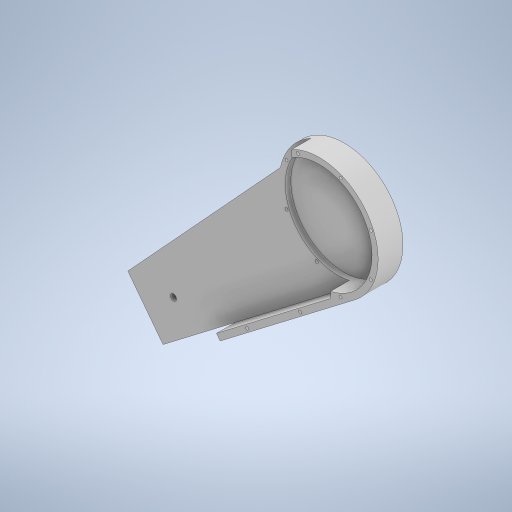
# Autodesk Inventor part: legparts_05
Saved by Autodesk Inventor 2024.3 (Build 283343000, 343)
## iProperties
Created: 2024-10-20
Part Number: legparts_05
Material: 一般
Document SubType Name: Modeling
Designer: 佐藤智貴
Density: 1 g/cm^3
Appearance: 既定
Author: 佐藤智貴
Autodesk Inventor part; units mm, degrees
ref_plane "YZ Plane" through (0, 0, 0) normal (1, 0, 0) x (0, 1, 0)
ref_plane "XZ Plane" through (0, 0, 0) normal (0, 1, 0) x (-1, 0, 0)
ref_plane "XY Plane" through (0, 0, 0) normal (0, 0, 1) x (1, 0, 0)
sketch "スケッチ1" plane through (0, 0, 0) normal (0, 0, 1) x (1, 0, 0)
  circle A0 centre (0, 0) radius 48.5
  circle A1 centre (0, 0) radius 46
  dimension "d0" = 97
  dimension "d1" = 92
  constraints: 2 centre point, 1 coincident
  measures "d0" diameter of A0
  measures "d1" diameter of A1
extrude "押し出し1" add sketch "スケッチ1" along normal blind 20.5 contours A0 | A1
sketch "スケッチ2" plane through (0, 0, 20.5) normal (0, 0, 1) x (1, 0, 0)
  circle A0 centre (0, 0) radius 46
  line L0 (0, 0) -> (0, 59.211017)
  line L1 (0, 0) -> (-21.860946, 52.776992)
  line L2 (0, 0) -> (27.822621, 47.858094)
  point P0 (-17.603438, 42.498458)
  point P1 (-42.498458, 17.603438)
  point P2 (-42.498458, -17.603438)
  point P3 (-17.603438, -42.498458)
  point P4 (17.603438, -42.498458)
  point P5 (42.498458, -17.603438)
  point P6 (42.498458, 17.603438)
  point P7 (17.603438, 42.498458)
  dimension "d4" = 92
  dimension "d5" = 22.5
  dimension "d8" = 360
  constraints: 6 end point, 1 coincident, 1 point on line, 1 vertical, 12 other
  measures "d5" angle of L1 L0
hole "穴1" at (-17.603438, 42.498458, 20.5) at (-42.498458, 17.603438, 20.5) at (-42.498458, -17.603438, 20.5) at (-17.603438, -42.498458, 20.5) at (17.603438, -42.498458, 20.5) at (42.498458, -17.603438, 20.5) at (42.498458, 17.603438, 20.5) at (17.603438, 42.498458, 20.5) direction (0, 0, -1) diameter 2.459 end through all
sketch "スケッチ3" plane through (0, 0, 20.5) normal (0, 0, 1) x (1, 0, 0)
  circle A0 centre (0, 0) radius 43.5
  dimension "d17" = 87
  constraints: 1 centre point, 1 coincident
  measures "d17" diameter of A0
extrude "押し出し2" cut sketch "スケッチ3" against normal blind 20
sketch "スケッチ4" plane through (0, 0, 0) normal (0, 0, -1) x (-1, 0, 0)
  line L0 (0, 0) -> (0, -80.557014)
  circle A0 centre (0, 0) radius 48.5
  line L1 (-29.457728, -38.529109) -> (145.313488, -172.151794)
  line L2 (29.457728, 38.529109) -> (204.228945, -95.093576)
  line L3 (145.313488, -172.151794) -> (204.228945, -95.093576)
  point P0 (29.457728, 38.529109)
  dimension "d21" = 48.5
  dimension "d23" = 97
  dimension "d24" = 220
  dimension "d25" = 220
  dimension "d56" = 52.6
  constraints: 8 end point, 1 perpendicular, 1 vertical, 2 other
  measures "d21" distance from line of L1 L0.start
  measures "d23" distance between parallel lines of L2 L1
  measures "d24" distance of L2.start L2.end
  measures "d25" distance of L1.start L1.end
  measures "d56" angle of L2 L0
extrude "押し出し3" add sketch "スケッチ4" against normal blind 5 contours A0 L2 L3 L1 L0 | L0 L1 A0
sketch "スケッチ5" plane through (0, 0, 5) normal (0, 0, 1) x (1, 0, 0)
  line L0 (-29.457728, 38.529109) -> (29.457728, -38.529109)
  line L1 (-204.228945, -95.093576) -> (-145.313488, -172.151794)
  line L2 (29.457728, -38.529109) -> (-145.313488, -172.151794)
  line L3 (-145.313488, -172.151794) -> (-204.228945, -95.093576)
  line L4 (-204.228945, -95.093576) -> (-29.457728, 38.529109)
  line L5 (-26.420849, 34.557036) -> (-201.192066, -99.065649)
  line L6 (26.420849, -34.557036) -> (-148.350367, -168.179721)
  line L7 (-200.256872, -92.056696) -> (-141.341415, -169.114915)
  circle A0 centre (0, 0) radius 48.5
  circle A1 centre (0, 0) radius 43.5
  point P0 (-116.843336, -28.282233)
  point P1 (-60.964759, -101.368378)
  point P2 (-57.92788, -105.340451)
  point P3 (-174.771217, -133.622685)
  point P4 (-170.799143, -130.585806)
  point P5 (-174.771217, -133.622685)
  point P6 (-43.459144, 21.530276)
  point P7 (9.382554, -47.583796)
  point P8 (-144.378294, -165.142842)
  point P9 (-197.219992, -96.02877)
  dimension "d29" = 5
  dimension "d30" = 5
  dimension "d32" = 5
  dimension "d33" = 5
  constraints: 14 end point, 6 midpoint, 6 point on line, 5 perpendicular, 1 collinear
  measures "d29" distance from line of point (-116.843, -28.282) L5
  measures "d30" distance of point (-60.965, -101.368) point (-57.928, -105.34)
  measures "d32" distance of point (-174.771, -133.623) point (-170.799, -130.586)
  measures "d33" radial gap between concentric circles of A0 A1
extrude "押し出し4" add sketch "スケッチ5" along normal blind 15.5 contours A0 L5 L7 L4 | L7 L5 L1 L4 | L7 L6 L1 L5 | L2 L7 L6 A0 | L7 L2 L1 L6
sketch "スケッチ6" plane through (0, 0, 20.5) normal (0, 0, 1) x (1, 0, 0)
  line L0 (-204.228945, -95.093576) -> (-145.313488, -172.151794)
  arc A0 (29.457728, -38.529109) -> (-29.457728, 38.529109) centre (0, 0) ccw
  line L1 (-29.457728, 38.529109) -> (-204.228945, -95.093576)
  line L2 (-145.313488, -172.151794) -> (29.457728, -38.529109)
  point P0 (-15.753516, -69.948744)
  point P1 (-71.632093, 3.137401)
  point P2 (-59.44632, -103.354415)
  point P3 (-115.324897, -30.26827)
  point P4 (-103.139124, -136.760086)
  point P5 (-159.017701, -63.673941)
  point P6 (-174.771217, -133.622685)
  point P7 (38.529109, 29.457728)
  point P8 (9.382554, -47.583796)
  dimension "d36" = 268.5
  dimension "d37" = 55
  dimension "d38" = 55
  dimension "d39" = 55
  dimension "d40" = 2.5
  dimension "d41" = 2.5
  dimension "d42" = 2.5
  dimension "d43" = 55
  dimension "d44" = 55
  dimension "d45" = 55
  dimension "d46" = 2.5
  dimension "d47" = 2.5
  dimension "d48" = 2.5
  constraints: 1 midpoint, 1 point on circle
  measures "d36" distance of point (-174.771, -133.623) point (38.529, 29.458)
  measures "d37" distance from line of L0 point (-159.018, -63.674)
  measures "d38" distance of point (-159.018, -63.674) point (-115.325, -30.268)
  measures "d39" distance of point (-115.325, -30.268) point (-71.632, 3.137)
  measures "d40" distance from line of L1 point (-71.632, 3.137)
  measures "d41" distance from line of L1 point (-115.325, -30.268)
  measures "d42" distance from line of L1 point (-159.018, -63.674)
  measures "d43" distance from line of L0 point (-103.139, -136.76)
  measures "d44" distance of point (-103.139, -136.76) point (-59.446, -103.354)
  measures "d45" distance of point (-15.754, -69.949) point (-59.446, -103.354)
  measures "d46" distance from line of L2 point (-15.754, -69.949)
  measures "d47" distance from line of L2 point (-59.446, -103.354)
  measures "d48" distance from line of L2 point (-103.139, -136.76)
hole "穴2" at (-15.753516, -69.948744, 20.5) at (-71.632093, 3.137401, 20.5) at (-59.44632, -103.354415, 20.5) at (-115.324897, -30.26827, 20.5) at (-103.139124, -136.760086, 20.5) at (-159.017701, -63.673941, 20.5) direction (0, 0, -1) diameter 2.459 end through all
sketch "スケッチ7" plane through (0, 0, 5) normal (0, 0, 1) x (1, 0, 0)
  line L0 (9.382554, -47.583796) -> (-144.378294, -165.142842)
  line L1 (-144.378294, -165.142842) -> (-197.219992, -96.02877)
  point P0 (0, 0)
  point P1 (-135.730252, -127.061201)
  dimension "d57" = 25
  dimension "d58" = 30
  measures "d57" distance from line of point (-135.73, -127.061) L0
  measures "d58" distance from line of L1 point (-135.73, -127.061)
hole "穴3" at (-135.730252, -127.061201, 5) direction (0, 0, -1) diameter 5 end through all
sketch "スケッチ8" plane through (0, 0, 5) normal (0, 0, 1) x (1, 0, 0)
  line L0 (-204.228945, -95.093576) -> (-29.457728, 38.529109)
  line L1 (29.457728, -38.529109) -> (-145.313488, -172.151794)
  line L2 (-204.228945, -95.093576) -> (-145.313488, -172.151794)
  line L3 (-145.313488, -172.151794) -> (-204.228945, -95.093576)
  line L4 (29.457728, -38.529109) -> (-145.313488, -172.151794)
  arc A0 (-43.459144, 21.530276) -> (9.382554, -47.583796) centre (0, 0) ccw
  line L5 (-43.459144, 21.530276) -> (-176.491161, -123.140956)
  line L6 (-197.219992, -96.02877) -> (-144.378294, -165.142842)
  line L7 (-47.512963, 9.734903) -> (-173.407433, -127.174304)
  dimension "d66" = 80
  dimension "d67" = 5
  constraints: 10 end point, 2 collinear, 2 point on line, 1 parallel, 1 perpendicular, 1 point on circle
  measures "d66" angle of L6 L5
  measures "d67" distance between parallel lines of L5 L7
extrude "押し出し5" add sketch "スケッチ8" along normal blind 10
sketch "スケッチ9" plane through (0, 0, 20.5) normal (0, 0, 1) x (1, 0, 0)
  circle A0 centre (0, 0) radius 48.5
  line L0 (-29.457728, 38.529109) -> (-204.228945, -95.093576)
  line L1 (-29.457728, 38.529109) -> (-204.228945, -95.093576)
  line L2 (-204.228945, -95.093576) -> (-144.905471, -172.685458)
  line L3 (-43.459144, 21.530276) -> (-179.92775, -126.878218)
  line L4 (-43.459144, 21.530276) -> (-176.491161, -123.140956)
  dimension "d70" = 97
  dimension "d71" = 80
  dimension "d72" = 0
  constraints: 6 end point, 2 collinear, 2 point on circle, 1 centre point, 1 coincident, 1 perpendicular, 1 point on line
  measures "d70" diameter of A0
  measures "d71" angle of L2 L3
  measures "d72" distance between parallel lines of L4 L3
sketch "スケッチ9 outline for 押し出し6" plane through (0, 0, 20.5) normal (0, 0, 1) x (1, 0, 0)
  line L0 (-179.92775, -126.878218) -> (-43.459144, 21.530276)
  line L1 (-204.228945, -95.093576) -> (-179.92775, -126.878218)
  line L2 (-29.457728, 38.529109) -> (-204.228945, -95.093576)
  arc A0 (-43.459144, 21.530276) -> (-29.457728, 38.529109) centre (0, 0) cw
extrude "押し出し6" cut sketch "スケッチ9 outline for 押し出し6" against normal through all
sketch "スケッチ10" plane through (0, 0, 20.5) normal (0, 0, 1) x (1, 0, 0)
  line L0 (-47.512963, 9.734903) -> (-173.407433, -127.174304)
  line L1 (-65.245855, -9.549472) -> (-68.329583, -5.516124)
  line L2 (-176.491161, -123.140956) -> (-179.92775, -126.878218)
  line L3 (-144.378294, -165.142842) -> (-173.407433, -127.174304)
  line L4 (-173.407433, -127.174304) -> (-176.527747, -123.093103)
  line L5 (-158.56619, -111.034574) -> (-161.649918, -107.001226)
  line L6 (-68.329583, -5.516124) -> (-161.649918, -107.001226)
  line L7 (-158.56619, -111.034574) -> (-65.245855, -9.549472)
  circle A0 centre (0, 0) radius 48.5
  line L8 (-43.459144, 21.530276) -> (-68.329583, -5.516124)
  line L9 (-47.512963, 9.734903) -> (-65.245855, -9.549472)
  line L10 (-158.56619, -111.034574) -> (-173.407433, -127.174304)
  line L11 (-144.378294, -165.142842) -> (-173.407433, -127.174304)
  line L12 (-179.92775, -126.878218) -> (-145.069701, -172.470655)
  line L13 (-144.378294, -165.142842) -> (9.382554, -47.583796)
  line L14 (-145.069701, -172.470655) -> (-81.516531, -123.880587)
  line L15 (-161.649918, -107.001226) -> (-179.92775, -126.878218)
  line L16 (-81.516531, -123.880587) -> (-84.797198, -119.589654)
  line L17 (9.382554, -47.583796) -> (9.382554, -42.583206)
  line L18 (-35.700709, 32.828485) -> (-32.020223, 29.444105)
  circle A1 centre (0, 0) radius 43.5
  circle A2 centre (0, 0) radius 43.5
  dimension "d75" = 97
  dimension "d78" = 80
  dimension "d79" = 87
  dimension "d80" = 5
  constraints: 30 end point, 6 collinear, 5 point on line, 4 parallel, 4 perpendicular, 2 centre point, 2 coincident, 1 point on circle, 1 vertical, 2 other
  measures "d75" diameter of A0
  measures "d78" distance of L12.end L14.end
  measures "d79" diameter of A2
  measures "d80" distance of L18.start L18.end
extrude "押し出し7" cut sketch "スケッチ10" against normal through all contours L0 L1 L8 A0 | L0 L5 L6 L1 | L0 L4 L15 L5 | L16 L14 L12 L2 L4 L3 L13
sketch "スケッチ11" plane through (0, 0, 20.5) normal (0, 0, 1) x (1, 0, 0)
  circle A0 centre (0, 0) radius 43.5
  circle A1 centre (0, 0) radius 48.5
  line L0 (-22.603438, 42.910775) -> (-22.603438, 37.16631)
  circle A2 centre (-17.603438, 42.498458) radius 1.2295
  arc A3 (-47.512963, 9.734903) -> (9.382554, -47.583796) centre (0, 0) ccw
  line L1 (9.382554, -47.583796) -> (9.382554, -42.476084)
  point P0 (-22.603438, 40.038542)
  dimension "d81" = 87
  dimension "d82" = 97
  dimension "d83" = 5
  constraints: 4 end point, 3 point on circle, 2 centre point, 2 vertical, 1 coincident, 1 midpoint
  measures "d81" diameter of A0
  measures "d82" diameter of A1
  measures "d83" horizontal distance of point (-22.603, 40.039) A2.centre
extrude "押し出し8" cut sketch "スケッチ11" against normal blind 15.5 contours A0 L1 A1 L0 picked at (-35.223195, -30.551112)
equation "\"d25\" = d24"
equation "\"d41\" = d40"
equation "\"d42\" = d41"
equation "\"d43\" = d37"
equation "\"d44\" = d43"
equation "\"d45\" = d44"
equation "\"d46\" = d40"
equation "\"d47\" = d46"
equation "\"d48\" = d46"
